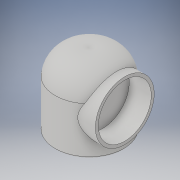
# Autodesk Inventor part: tete
Saved by Autodesk Inventor 2018 (Build 220112000, 112)
## iProperties
Created: 2018-04-09
Part Number: tete
Material: Generic
Document SubType Name: Modeling
Designer: usrvauban02
Density: 1 g/cm^3
Appearance: Default
Author: usrvauban02
## iProperties of the stored document Part1_3DPrint.ipt
Created: 2018-04-09
Part Number: Part1_3DPrint
Material: Generic
Document SubType Name: Modeling
Designer: usrvauban02
Density: 1 g/cm^3
Appearance: Default
Author: usrvauban02
Autodesk Inventor part; units mm, degrees
ref_plane "YZ Plane" through (0, 0, 0) normal (1, 0, 0) x (0, 1, 0)
ref_plane "XZ Plane" through (0, 0, 0) normal (0, 1, 0) x (-1, 0, 0)
ref_plane "XY Plane" through (0, 0, 0) normal (0, 0, 1) x (1, 0, 0)
sketch "Sketch1" plane through (0, 0, 0) normal (0, 0, 1) x (1, 0, 0)
  line L0 (0, 0) -> (60, 0)
  line L1 (0, 126.1861) -> (0, 150)
  line L2 (0, 18.2402) -> (0, 0)
  line L3 (0, 126.1861) -> (0, 18.2402)
  line L4 (70, 7.0021) -> (70, 100.5361)
  arc A0 (70, 100.5361) -> (0, 150) centre (14.4108, 96.1307) ccw
  arc A1 (60, 0) -> (70, 7.0021) centre (57.6261, 14.0321) ccw
  point P0 (84.7515, 38.5438)
  dimension "d1" = 60
  dimension "d2" = 150
  dimension "d22" = 10
  constraints: 10 end point, 4 point on circle, 2 centre point, 2 vertical, 1 collinear, 1 horizontal
  measures "d1" distance of L0.start L0.end
  measures "d2" distance of L0.start L1.end
  measures "d22" horizontal distance of L0.end L4.start
revolve "Revolution1" add sketch "Sketch1" angle 360 about axis through (0, 126.1861, 0) along (0, -1, 0)
sketch "Sketch2" plane through (0, 0, 0) normal (1, 0, 0) x (0, 1, 0)
  line L0 (0, 75) -> (0, -75) projected
  circle A0 centre (75, 0) radius 60
  point P0 (0, 0)
  point P1 (150, 0)
  dimension "d4" = 120
  dimension "d25" = 75
  constraints: 1 centre point
  measures "d4" diameter of A0
  measures "d25" distance from line of A0.centre L0
extrude "Extrusion1" add sketch "Sketch2" along normal blind 72
hole "Hole1" at (72, 75, 0) direction (-1, 0, 0) diameter 108 depth 45
body "Solid1"
